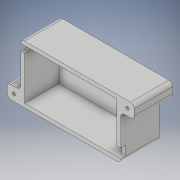
# Autodesk Inventor part: Крышка Модуля БП
Saved by Autodesk Inventor 2019 (Build 230136000, 136)
## iProperties
Created: 2018-07-03
Part Number: Крышка Модуля БП
Material: Типовые
Document SubType Name: Modeling
Designer: rossolov
Density: 1 g/cm^3
Appearance: По умолчанию
Author: rossolov
Autodesk Inventor part; units mm, degrees
ref_plane "YZ Plane" through (0, 0, 0) normal (1, 0, 0) x (0, 1, 0)
ref_plane "XZ Plane" through (0, 0, 0) normal (0, 1, 0) x (-1, 0, 0)
ref_plane "XY Plane" through (0, 0, 0) normal (0, 0, 1) x (1, 0, 0)
sketch "Эскиз1" plane through (0, 0, 0) normal (0, 0, 1) x (1, 0, 0)
  line L0 (-9.5803, -22.5479) -> (42.4197, -22.5479)
  line L1 (42.4197, -22.5479) -> (42.4197, 7.4521)
  line L2 (42.4197, 7.4521) -> (-9.5803, 7.4521)
  line L3 (-9.5803, 7.4521) -> (-9.5803, -22.5479)
  constraints: 8 end point, 2 parallel, 1 horizontal, 1 perpendicular
extrude "Выдавливание1" add sketch "Эскиз1" along normal blind 2
sketch "Эскиз2" plane through (0, 0, 2) normal (0, 0, 1) x (1, 0, 0)
  line L0 (-9.5803, 7.4521) -> (-9.5803, -22.5479) projected
  line L1 (-9.5803, -22.5479) -> (42.4197, -22.5479) projected
  line L2 (-9.5803, 7.4521) -> (42.4197, 7.4521)
  line L3 (42.4197, 7.4521) -> (42.4197, -22.5479)
  line L4 (42.4197, -22.5479) -> (-9.5803, -22.5479)
  line L5 (-9.5803, -22.5479) -> (-9.5803, 7.4521)
  line L6 (42.4197, 7.4521) -> (-9.5803, 7.4521) projected
  line L7 (-9.5803, 7.4521) -> (-7.5803, 7.4521)
  line L8 (42.4197, -22.5479) -> (40.4197, -22.5479)
  line L9 (40.4197, -20.5479) -> (-7.5803, -20.5479)
  line L10 (-7.5803, -20.5479) -> (-7.5803, 5.4521)
  line L11 (-7.5803, 5.4521) -> (40.4197, 5.4521)
  line L12 (40.4197, 5.4521) -> (40.4197, -20.5479)
  point P0 (0, 0)
  constraints: 20 end point, 4 parallel, 2 horizontal, 2 perpendicular, 2 point on line
extrude "Выдавливание2" add sketch "Эскиз2" along normal blind 18
sketch "Эскиз6" plane through (0, 0, 0) normal (0, 0, -1) x (-1, 0, 0)
  line L0 (9.5803, -22.5479) -> (-42.4197, -22.5479) projected
  line L1 (9.5803, -22.5479) -> (16.5803, -22.5479)
  line L2 (16.5803, -22.5479) -> (16.5803, -15.5479)
  line L3 (16.5803, -15.5479) -> (9.5803, -15.5479)
  line L4 (9.5803, -15.5479) -> (9.5803, -22.5479)
  line L5 (-42.4197, 7.4521) -> (-49.4197, 7.4521)
  line L6 (-49.4197, 7.4521) -> (-49.4197, 0.4521)
  line L7 (-49.4197, 0.4521) -> (-42.4197, 0.4521)
  line L8 (-42.4197, 0.4521) -> (-42.4197, 7.4521)
  point P0 (0, 0)
  dimension "d22" = 7
  dimension "d23" = 7
  dimension "d24" = 7
  dimension "d25" = 7
  constraints: 16 end point, 4 parallel, 2 horizontal, 2 perpendicular
  measures "d22" distance of L3.end L2.end
  measures "d23" distance of L2.end L1.end
  measures "d24" distance of L7.end L6.end
  measures "d25" distance of L6.end L5.end
extrude "Выдавливание5" add sketch "Эскиз6" against normal blind 20
sketch "Эскиз7" plane through (42.4197, -22.5479, 20) normal (1, 0, 0) x (0, 0, -1)
  line L0 (0, 2) -> (0, 28) projected
  line L1 (0, 2) -> (2.5, 2)
  line L2 (2.5, 2) -> (2.5, 7)
  line L3 (2.5, 7) -> (0, 7)
  line L4 (0, 7) -> (0, 2)
  point P0 (20, 22.5479)
  dimension "d28" = 2.5
  dimension "d29" = 5
  constraints: 8 end point, 2 parallel, 1 horizontal, 1 perpendicular
  measures "d28" distance of L3.end L2.end
  measures "d29" distance of L2.end L1.end
extrude "Выдавливание6" cut sketch "Эскиз7" against normal blind 2
sketch "Эскиз8" plane through (-9.5803, 7.4521, 0) normal (-1, 0, 0) x (0, 0, 1)
  line L0 (2, -2) -> (20, -2) projected
  line L1 (20, -2) -> (18.25, -2)
  line L2 (16.5, -3.75) -> (16.5, -3.75)
  line L3 (18.25, -5.5) -> (20, -5.5)
  line L4 (20, -5.5) -> (20, -2)
  arc A0 (18.25, -2) -> (16.5, -3.75) centre (18.25, -3.75) ccw
  arc A1 (16.5, -3.75) -> (18.25, -5.5) centre (18.25, -3.75) ccw
  point P0 (0, -7.4521)
  point P1 (16.5, -5.5)
  point P2 (16.5, -2)
  dimension "d32" = 3.5
  dimension "d33" = 3.5
  dimension "d34" = 1.75
  constraints: 8 end point, 4 point on circle, 4 point on line, 4 tangent, 2 centre point, 2 parallel, 1 concentric, 1 horizontal, 1 perpendicular
  measures "d32" distance of L3.end point (16.5, -5.5)
  measures "d33" distance of point (16.5, -5.5) point (16.5, -2)
  measures "d34" radius of A0
extrude "Выдавливание7" cut sketch "Эскиз8" against normal blind 2
fillet "Сопряжение1" radius 0.5 2 edges at (41.4197, -15.5479, 17.5) (41.4197, -20.5479, 17.5)
fillet "Сопряжение2" radius 2 8 edges at (42.4197, 0.4521, 10) (49.4197, 0.4521, 10) (49.4197, 7.4521, 10) (-9.5803, 7.4521, 10) (-16.5803, -22.5479, 10) (-16.5803, -15.5479, 10) (42.4197, -22.5479, 10) (-9.5803, -15.5479, 10)
sketch "Эскиз9" plane through (0, 0, 20) normal (0, 0, 1) x (1, 0, 0)
  circle A0 centre (-13.0803, -19.0479) radius 0.85
  point P0 (0, 0)
  point P1 (-16.5803, -17.5479)
  point P2 (-14.5803, -15.5479)
  dimension "d39" = 1.7
  constraints: 1 centre point
  measures "d39" diameter of A0
sketch "Эскиз10" plane through (0, 0, 20) normal (0, 0, 1) x (1, 0, 0)
  arc A0 (47.4197, 0.4521) -> (49.4197, 2.4521) centre (47.4197, 2.4521) ccw projected
  circle A1 centre (45.9197, 3.9521) radius 0.85
  point P0 (0, 0)
  dimension "d41" = 1.7
  constraints: 1 centre point
  measures "d41" diameter of A1
extrude "Выдавливание8" cut sketch "Эскиз9" against normal blind 15
extrude "Выдавливание9" cut sketch "Эскиз10" against normal blind 15
